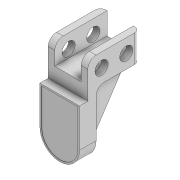
# Autodesk Inventor part: Holder of gripper
Saved by Autodesk Inventor 2020.3 (Build 243373010, 373A)
## iProperties
Created: 2021-05-15
Part Number: Holder of gripper
Material: Generic
Document SubType Name: Modeling
Designer: marti
Density: 1 g/cm^3
Appearance: Default
Author: marti
Autodesk Inventor part; units mm, degrees
ref_plane "YZ Plane" through (0, 0, 0) normal (1, 0, 0) x (0, 1, 0)
ref_plane "XZ Plane" through (0, 0, 0) normal (0, 1, 0) x (-1, 0, 0)
ref_plane "XY Plane" through (0, 0, 0) normal (0, 0, 1) x (1, 0, 0)
sketch "Sketch1" plane through (0, 0, 0) normal (0, 0, 1) x (1, 0, 0)
  arc A0 (-18, 0) -> (18, 0) centre (0, 0) ccw
  line L0 (-18, 0) -> (-18, 35)
  line L1 (18, 0) -> (18, 35)
  line L2 (-18, 35) -> (18, 35)
  dimension "d0" = 36
  dimension "d2" = 35
  constraints: 6 end point, 2 point on circle, 2 tangent, 2 vertical, 1 centre point, 1 coincident, 1 horizontal
  measures "d0" diameter of A0
  measures "d2" distance from line of point (0, 0) L2
extrude "Extrusion1" add sketch "Sketch1" against normal mid plane 15
sketch "Sketch2" plane through (0, 0, 0) normal (1, 0, 0) x (0, 1, 0)
  line L0 (35, -7.5) -> (0, -7.5) projected
  line L1 (35, -7.5) -> (35, 7.5) projected
  arc A0 (42.5, -15) -> (35, -7.5) centre (35, -15) ccw
  line L2 (42.5, -47.5) -> (42.5, -15)
  line L3 (42.5, -47.5) -> (67.5, -47.5)
  line L4 (67.5, -47.5) -> (67.5, -7.5)
  line L5 (60, 0) -> (35, 0)
  arc A1 (67.5, -7.5) -> (60, 0) centre (60, -7.5) ccw
  point P0 (0, 0)
  dimension "d10" = 40
  dimension "d11" = 25
  dimension "d12" = 15
  constraints: 8 end point, 4 point on circle, 3 tangent, 2 centre point, 2 vertical, 1 horizontal, 1 midpoint
  measures "d10" distance from line of L0 L2.start
  measures "d11" distance of L2.start L3.end
  measures "d12" diameter of A1
extrude "Extrusion2" add sketch "Sketch2" along normal mid plane 36
sketch "Sketch3" plane through (0, 0, 0) normal (1, 0, 0) x (0, 1, 0)
  line L0 (42.5, -47.5) -> (67.5, -47.5) projected
  line L1 (-18, -7.5) -> (0, -7.5) projected
  line L2 (42.5, -47.5) -> (-18, -7.5)
  line L3 (35, -7.5) -> (0, -7.5) projected
  arc A0 (42.5, -15) -> (35, -7.5) centre (35, -15) ccw projected
  line L4 (42.5, -15) -> (42.5, -47.5) projected
  point P0 (0, 0)
  constraints: 2 end point
extrude "Extrusion3" add sketch "Sketch3" along normal mid plane 15
delete faces "Delete Face1" heal yes whole lump no faces at (-6.6957, -17.2098, -7.5) (6.6957, -17.2098, -7.5)
fillet "Fillet1" radius 2 6 edges at (-7.5, 40.3033, -9.6967) (-7.5, 42.5, -31.25) (-7.5, 9.3185, -7.5) (7.5, 42.5, -31.25) (7.5, 9.3185, -7.5) (7.5, 40.3033, -9.6967)
sketch "Sketch5" plane through (0, 0, 0) normal (1, 0, 0) x (0, 1, 0)
  line L0 (47.5, -54.8971) -> (47.5, 0)
  line L1 (67.5, -47.5) -> (67.5, -7.5) projected
  line L2 (0, -7.5) -> (0, 7.5) projected
  line L3 (35, -7.5) -> (0, -7.5) projected
  arc A0 (42.5, -15) -> (35, -7.5) centre (35, -15) ccw projected
  line L4 (42.5, -15) -> (42.5, -47.5) projected
  line L5 (42.5, -47.5) -> (67.5, -47.5) projected
  line L6 (67.5, -47.5) -> (67.5, -7.5) projected
  arc A1 (67.5, -7.5) -> (60, 0) centre (60, -7.5) ccw projected
  line L7 (60, 0) -> (35, 0) projected
  line L8 (35, 0) -> (35, 7.5) projected
  line L9 (0, 7.5) -> (35, 7.5) projected
  point P0 (0, 0)
  point P1 (47.5, -47.5)
  dimension "d21" = 20
  constraints: 2 end point, 1 midpoint, 1 vertical
  measures "d21" distance between parallel lines of L1 L0
extrude "Extrusion5" cut sketch "Sketch5" against normal mid plane 24 contours L0 L7 A1 L1 L5
sketch "Sketch6" plane through (0, 0, 7.5) normal (0, 0, 1) x (1, 0, 0)
  arc A0 (-18, 0) -> (18, 0) centre (0, 0) ccw projected
  line L0 (18, 0) -> (18, 35) projected
  line L1 (18, 35) -> (-18, 35) projected
  line L2 (-18, 35) -> (-18, 0) projected
  arc A1 (-16.5, 0) -> (16.5, 0) centre (0, 0) ccw
  line L3 (-16.5, 0) -> (-16.5, 33.5)
  line L4 (-16.5, 33.5) -> (16.5, 33.5)
  line L5 (16.5, 33.5) -> (16.5, 0)
  dimension "d24" = 1.5
  constraints: 6 end point, 2 point on circle, 1 centre point, 3 other
  measures "d24" radial gap between concentric circles of A0 A1
extrude "Extrusion6" cut sketch "Sketch6" against normal blind 0.25 contours L3 L4 L5 A1
fillet "Fillet2" radius 5 2 edges at (-18, 55, -47.5) (18, 55, -47.5)
sketch "Sketch7" plane through (-18, 35, 0) normal (-1, 0, 0) x (0, 0, 1)
  line L0 (-42.5, 7.5) -> (-42.5, 32.5) projected
  line L1 (-42.5, 7.5) -> (-15, 7.5) projected
  arc A0 (-7.5, 0) -> (-15, 7.5) centre (-15, 0) ccw projected
  line L2 (-7.5, -35) -> (-7.5, 0) projected
  line L3 (7.5, -35) -> (-7.5, -35) projected
  line L4 (7.5, 0) -> (7.5, -35) projected
  line L5 (0, 0) -> (7.5, 0) projected
  line L6 (0, 0) -> (0, 25) projected
  arc A1 (0, 25) -> (-7.5, 32.5) centre (-7.5, 25) ccw projected
  line L7 (-7.5, 32.5) -> (-42.5, 32.5) projected
  circle A2 centre (-12.5, 20) radius 6
  line L8 (-47.5, 32.5) -> (-47.5, 7.5) projected
  circle A3 centre (-35, 20) radius 6
  point P0 (0, -35)
  point P1 (-47.5, 20)
  dimension "d28" = 25
  dimension "d29" = 12
  dimension "d30" = 47.5
  dimension "d31" = 12.5
  dimension "d32" = 12
  dimension "d33" = 12.5
  constraints: 2 centre point, 2 horizontal alignment, 1 midpoint
  measures "d28" distance between parallel lines of L7 L1
  measures "d29" diameter of A2
  measures "d30" distance between parallel lines of L8 L6
  measures "d31" distance from line of L6 A2.centre
  measures "d32" diameter of A3
  measures "d33" distance from line of L8 A3.centre
extrude "Extrusion7" cut sketch "Sketch7" against normal through all contours A2 | A3
body "Solid1"
